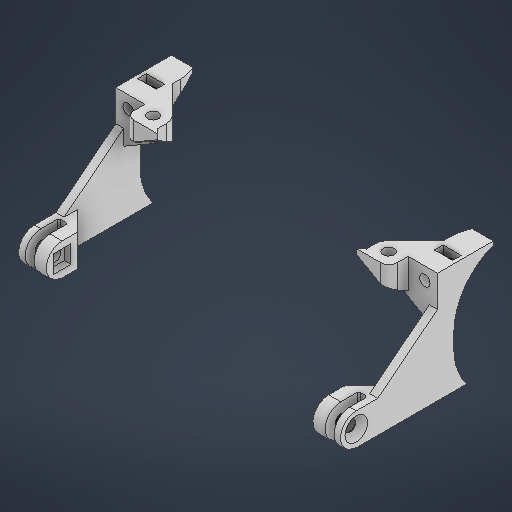
# Autodesk Inventor part: body-main
Saved by Autodesk Inventor 2025 (Build 290162000, 162)
## iProperties
Created: 2024-10-19
Part Number: body-main
Material: Všeobecné
Document SubType Name: Modeling
Designer: Simak
Density: 1 g/cm^3
Appearance: Výchozí
Author: Simak
Autodesk Inventor part; units mm, degrees
ref_plane "YZ Plane" through (0, 0, 0) normal (1, 0, 0) x (0, 1, 0)
ref_plane "XZ Plane" through (0, 0, 0) normal (0, 1, 0) x (-1, 0, 0)
ref_plane "XY Plane" through (0, 0, 0) normal (0, 0, 1) x (1, 0, 0)
sketch "Náčrt1" plane through (0, 0, 0) normal (1, 0, 0) x (0, 1, 0)
  circle A0 centre (5, 0) radius 5 construction
  line L0 (10, 0) -> (10, -6.8) construction
  line L1 (9.85, -6.6099) -> (24.35, -24.9833)
  line L2 (0, 0) -> (0, -39.0132)
  line L3 (24.35, -24.9833) -> (34, -24.9833)
  line L4 (34, -24.9833) -> (34, -42.1726)
  circle A1 centre (13.5, -48.5) radius 16.5 construction
  line L5 (10, -5) -> (0, -5) construction
  line L6 (15.5, -30) -> (11.5, -30)
  arc A2 (11.5, -30) -> (0, -34.0086) centre (11.5, -48.5) ccw
  arc A3 (32.8843, -42.1726) -> (15.5, -30) centre (15.5, -48.5) ccw
  line L7 (32.8843, -42.1726) -> (34, -45.238) construction
  line L8 (32.8843, -42.1726) -> (34, -42.1726)
  circle A4 centre (5, 0) radius 4.85
  line L9 (9.85, 0) -> (9.85, -6.6099)
  line L10 (0, 0) -> (0.2955, 1.1791)
  point P0 (13.5, -65)
  point P1 (13.5, -30)
  dimension "d0" = 10
  dimension "d1" = 33
  dimension "d3" = 3
  dimension "d4" = 65
  dimension "d5" = 128.28
  dimension "d6" = 34
  dimension "d7" = 9.65
  dimension "d8" = 6.8
  dimension "d9" = 4
  dimension "d10" = 2
  dimension "d11" = 18.5
  dimension "d13" = 70
  dimension "d14" = 9.7
  constraints: 23 end point, 10 point on circle, 8 tangent, 7 point on line, 5 centre point, 4 perpendicular, 2 horizontal, 2 vertical, 2 vertical alignment, 1 coincident, 1 equal radius, 1 midpoint
  measures "d0" diameter of A0
  measures "d1" diameter of A1
  measures "d3" distance edge to line of A1 L2
  measures "d4" vertical distance of A1.start A0.centre
  measures "d5" angle of L1 L5
  measures "d6" distance between parallel lines of L4 L2
  measures "d7" distance of L1.end L3.end
  measures "d8" vertical distance of A0.centre L0.end
  measures "d9" distance of L6.start L6.end
  measures "d10" distance edge to line of A1 L6
  measures "d11" radius of A2
  measures "d13" angle of L7 L3
  measures "d14" diameter of A4
extrude "Vysunutí1" add sketch "Náčrt1" along normal blind 49.5
sketch "Náčrt2" plane through (0, 0, -34.0086) normal (0, -1, 0) x (1, 0, 0)
  line L0 (0, 38.8586) -> (49.5, 38.8586) projected
  line L1 (49.5, 34.0086) -> (49.5, 38.8586) projected
  line L2 (49.5, 34.0086) -> (49.5, 35.1877) projected
  line L3 (49.5, 35.1877) -> (49.5, 34.0086) projected
  line L4 (49.5, 34.0086) -> (49.5, 0) projected
  line L5 (49.5, 0) -> (49.5, 4.0086) projected
  line L6 (49.5, 4.0086) -> (49.5, -8.164) projected
  line L7 (49.5, -8.164) -> (49.5, 9.0253) projected
  line L8 (49.5, 9.0253) -> (49.5, 27.3987) projected
  line L9 (49.5, 27.3987) -> (49.5, 34.0086) projected
  line L10 (0, 34.0086) -> (0, 35.1877) projected
  line L11 (0, 27.3987) -> (0, 34.0086) projected
  line L12 (0, 9.0253) -> (0, 27.3987) projected
  line L13 (0, -8.164) -> (0, 9.0253) projected
  line L14 (0, 4.0086) -> (0, -8.164) projected
  line L15 (0, 0) -> (0, 4.0086) projected
  line L16 (0, 34.0086) -> (0, 0) projected
  line L17 (0, 35.1877) -> (0, 34.0086) projected
  line L18 (0, 34.0086) -> (0, 38.8586) projected
  line L19 (0, -8.164) -> (49.5, -8.164) projected
  line L20 (47, 38.8586) -> (47, -8.164)
  dimension "d17" = 2.5
  constraints: 2 end point, 2 point on line, 1 perpendicular
  measures "d17" distance between parallel lines of L8 L20
extrude "Vysunutí2" cut sketch "Náčrt2" against normal through all contours L0 L20 L19 L13 L12 L11 L10 L18
sketch "Náčrt3" plane through (49.5, 0, -34.0086) normal (0, -1, 0) x (1, 0, 0)
  line L0 (-2.5, 38.8586) -> (0, 38.8586) projected
  line L1 (0, 34.0086) -> (0, 35.1877) projected
  line L2 (0, 35.1877) -> (0, 34.0086) projected
  line L3 (0, 34.0086) -> (0, 0) projected
  line L4 (0, 0) -> (0, 4.0086) projected
  line L5 (0, 4.0086) -> (0, -8.164) projected
  line L6 (0, -8.164) -> (0, 9.0253) projected
  line L7 (0, 9.0253) -> (0, 27.3987) projected
  line L8 (0, 27.3987) -> (0, 34.0086) projected
  line L9 (0, 34.0086) -> (0, 38.8586) projected
  line L10 (-2.5, 0) -> (-2.5, 4.0086) projected
  line L11 (-2.5, 34.0086) -> (-2.5, 0) projected
  line L12 (-2.5, 35.1877) -> (-2.5, 34.0086) projected
  line L13 (-2.5, 34.0086) -> (-2.5, 35.1877) projected
  line L14 (-2.5, 27.3987) -> (-2.5, 34.0086) projected
  line L15 (-2.5, 9.0253) -> (-2.5, 27.3987) projected
  line L16 (-2.5, -8.164) -> (-2.5, 9.0253) projected
  line L17 (-2.5, 4.0086) -> (-2.5, -8.164) projected
  line L18 (-2.5, 34.0086) -> (-2.5, 38.8586) projected
  line L19 (-2.5, -8.164) -> (0, -8.164) projected
  line L20 (-2, 38.8586) -> (-2, 29.0086)
  line L21 (-49.5, 29.1586) -> (-49.5, 38.8586) projected
  line L22 (-49.5, 29.0086) -> (-49.5, 39.0086) construction
  line L23 (-2, 29.0086) -> (-4.75, 29.0086)
  line L24 (-4.75, 29.0086) -> (-4.75, 38.8586)
  line L25 (-6.5, 38.8586) -> (-6.5, 27.2231)
  line L26 (-4.75, 38.8586) -> (-6.5, 38.8586)
  line L27 (-6.5, 27.2231) -> (-2.5, 23.2231)
  line L28 (-2, 29.0086) -> (-2.5, 28.5086)
  line L29 (-4.75, 29.0086) -> (-4.25, 28.5086)
  line L30 (-4.25, 28.5086) -> (-2.5, 28.5086)
  point P0 (-49.5, 34.0086)
  point P1 (-49.5, 34.0086)
  point P2 (-2.5, 29.0086)
  dimension "d20" = 2
  dimension "d21" = 2.75
  dimension "d22" = 6.5
  dimension "d23" = 45
  dimension "d24" = 2.5
  dimension "d25" = 45
  constraints: 18 end point, 3 horizontal, 3 perpendicular, 3 point on line, 2 horizontal alignment, 1 vertical
  measures "d20" distance between parallel lines of L9 L20
  measures "d21" distance of L20.end L23.end
  measures "d22" distance between parallel lines of L3 L25
  measures "d23" angle of L15 L27
  measures "d24" distance from line of L23.end L27
  measures "d25" angle of L14 L28
extrude "Vysunutí3" cut sketch "Náčrt3" against normal up to surface (9.85 mm away) contours L0 L20 L23 L11 L12 L18 | L28 L11 L23
extrude "Vysunutí4" add sketch "Náčrt3" against normal up to surface (9.85 mm away) contours L11 L27 L25 L26 L24 L29 L30
sketch "Náčrt4" plane through (49.5, 0, 0) normal (1, 0, 0) x (0, 0, -1)
  line L0 (5, 9.85) -> (-4.85, 9.85) projected
  line L1 (-4.85, 0) -> (-4.85, 9.85) projected
  line L2 (5, 0) -> (-4.85, 0) projected
  line L3 (5, 0) -> (5, 9.85) projected
  arc A0 (0, 9.85) -> (-1.1791, 0.2955) centre (0, 5) ccw projected
  line L4 (-1.1791, 0.2955) -> (0, 0) projected
  line L5 (0, 0) -> (34.0086, 0) projected
  arc A1 (30, 11.5) -> (34.0086, 0) centre (48.5, 11.5) ccw projected
  line L6 (30, 11.5) -> (30, 15.5) projected
  arc A2 (42.1726, 32.8843) -> (30, 15.5) centre (48.5, 15.5) ccw projected
  line L7 (42.1726, 32.8843) -> (42.1726, 34) projected
  line L8 (42.1726, 34) -> (24.9833, 34) projected
  line L9 (24.9833, 34) -> (24.9833, 24.35) projected
  line L10 (24.9833, 24.35) -> (6.6099, 9.85) projected
  line L11 (6.6099, 9.85) -> (0, 9.85) projected
  point P0 (-4.85, 5)
extrude "Vysunutí5" cut sketch "Náčrt4" against normal through all contours A0 L1 L0 | A0 L4 L2 L1
sketch "Náčrt5" plane through (49.5, 0, 0) normal (1, 0, 0) x (0, 0, -1)
  arc A0 (0, 9.85) -> (-1.1791, 0.2955) centre (0, 5) ccw projected
  point P0 (0, 0)
  constraints: 1 coincident
hole "Díra1" at (49.5, 5, 0) direction (-1, 0, 0) diameter 3.4 end through all countersink diameter 7 countersink angle 90
sketch "Náčrt6" plane through (43, 0, -6.7855) normal (-1, 0, 0) x (0, 0, 1)
  line L0 (4.0355, 7.75) -> (9.5355, 7.75)
  line L1 (9.5355, 7.75) -> (9.5355, 2.25)
  line L2 (9.5355, 2.25) -> (4.0355, 2.25)
  line L3 (4.0355, 2.25) -> (4.0355, 7.75)
  circle A0 centre (6.7855, 5) radius 3.5 projected
  line L4 (4.0355, 7.75) -> (6.7855, 5) construction
  line L5 (6.7855, 5) -> (9.5355, 7.75) construction
  line L6 (4.0355, 2.25) -> (6.7855, 5) construction
  circle A1 centre (6.7855, 5) radius 1.7 projected
  arc A2 (7.9646, 0.2955) -> (6.7855, 9.85) centre (6.7855, 5) ccw projected
  line L7 (6.7855, 9.85) -> (0, 9.85) projected
  line L8 (0, 0) -> (0, 9.85) projected
  line L9 (6.7855, 0) -> (0, 0) projected
  line L10 (6.7855, 0) -> (7.9646, 0.2955) projected
  dimension "d39" = 5.5
  constraints: 14 end point, 5 perpendicular, 2 parallel, 1 horizontal
  measures "d39" distance of L1.end L2.end
extrude "Vysunutí6" add sketch "Náčrt6" along normal blind 2 contours A0 L0 | L3 A0 | A0 L1 | L2 A0 | L10 L9 L8 L7 A2
sketch "Náčrt7" plane through (49.5, 9.85, 0) normal (0, 1, 0) x (1, 0, 0)
  line L0 (-8.5, 0) -> (-8.5, 6.7855) projected
  line L1 (-6.5, 6.7855) -> (-8.5, 6.7855) projected
  line L2 (-6.5, 6.7855) -> (-2.5, 10.7855) projected
  line L3 (-6.5, 6.7855) -> (-8.5, 4.7855)
  point P0 (-49.5, 0)
  constraints: 2 end point, 1 collinear, 1 point on line
extrude "Vysunutí7" cut sketch "Náčrt7" against normal through all
sketch "Náčrt8" plane through (49.5, 24.35, -24.9833) normal (0, 0, 1) x (1, 0, 0)
  circle A0 centre (-3.875, 5.775) radius 1.65
  line L0 (0, 9.65) -> (0, 0) projected
  line L1 (-2.5, 9.65) -> (0, 9.65) projected
  circle A1 centre (-3.875, 5.775) radius 3.875
  line L2 (-7.75, 3.85) -> (-2.5, -0.1301)
  line L3 (-2.5, 9.65) -> (-2.5, 0) projected
  line L4 (-2.5, 0) -> (-2.5, -14.5) projected
  line L5 (-3.875, 9.65) -> (-2.5, 9.65)
  line L6 (-7.75, 3.85) -> (-7.75, 5.775)
  point P0 (-49.5, -24.35)
  point P1 (-2.5, 9.3978)
  point P2 (0, 5.775)
  point P3 (-2.5, 2.1522)
  point P4 (-6.216, 2.6871)
  point P5 (-6.216, 2.6871)
  dimension "d44" = 3.875
  dimension "d45" = 3.875
  dimension "d46" = 3.3
  dimension "d77" = 5.8
  constraints: 6 end point, 4 tangent, 2 centre point, 2 point on circle, 1 coincident, 1 horizontal alignment, 1 point on line, 1 vertical, 1 vertical alignment
  measures "d44" distance from line of L0 A0.centre
  measures "d45" distance from line of L1 A0.centre
  measures "d46" diameter of A0
  measures "d77" distance from line of L2.start L1
extrude "Vysunutí8" add sketch "Náčrt8" against normal up to surface contours L3 A0 | A0 L3 A1 | A1 L5 L3 | L3 L4 L2 A1 | L2 L6 A1 round surface about axis through (0, 15.5, -48.5) along (1, 0, 0) radius 18.5 far side no picked at (-3.5043, 5.7082) picked at (-6.0124, 3.508)
extrude "Vysunutí9" cut sketch "Náčrt8" against normal through all contours A0 L3 | L3 A0
sketch "Náčrt9" plane through (49.5, 34, -24.9833) normal (0, 1, 0) x (1, 0, 0)
  line L0 (-5.525, 0) -> (-5.525, 12.1871) projected
  line L1 (-2.225, 0) -> (-2.225, 12.1871) projected
  line L2 (-7.75, 0) -> (-7.75, 12.1871) projected
  spline S0 degree 7 poles (-3.875, 23.5167) (-4.2595, 22.6766) (-4.6432, 21.8383) (-5.0232, 20.9998) (-5.3966, 20.1601) (-5.7592, 19.3189) (-6.1055, 18.4772) (-6.6646, 17.0171) (-6.8881, 16.3994) (-7.0958, 15.7818) (-7.284, 15.1633) (-7.4474, 14.545) (-7.5778, 13.9297) (-7.687, 13.1584) (-7.707, 12.9949) (-7.7236, 12.8319) (-7.7365, 12.6695) (-7.7454, 12.5078) (-7.75, 12.3469) (-7.75, 12.1871) knots 0 0 0 0 0 0 0 0 0.51596 0.51596 0.51596 0.51596 0.51596 0.51596 0.897167 0.897167 0.897167 0.897167 0.897167 0.897167 1 1 1 1 1 1 1 1 projected
  line L3 (-2.5, 23.5167) -> (-3.875, 23.5167) projected
  line L4 (-2.5, 17.1893) -> (-2.5, 23.5167) projected
  line L5 (-2.5, 17.1893) -> (-2.5, 12.1871)
  line L6 (-7.75, 12.1871) -> (-2.5, 12.1871)
  line L7 (-2.5, 17.1893) -> (-6.5956, 17.1893)
  point P0 (-49.5, -24.9833)
  point P1 (-5.8125, 8.8451)
  point P2 (-2.5, 8.6438)
  constraints: 6 end point, 2 horizontal, 1 vertical, 2 other
extrude "Vysunutí10" cut sketch "Náčrt9" against normal up to next contours L3 L4 L7 S0
ref_plane "Pracovní rovina1" through (49.5, 24.35, -30.7333) normal (0, 0, 1) x (1, 0, 0)
sketch "Náčrt10" plane through (49.5, 24.35, -30.7333) normal (0, 0, 1) x (1, 0, 0)
  arc A0 (-3.875, 9.65) -> (-7.75, 5.775) centre (-3.875, 5.775) ccw projected
  line L0 (-3.875, 9.65) -> (0, 9.65) projected
  circle A1 centre (-3.875, 5.775) radius 1.65 projected
  line L1 (-2.5, 0) -> (-2.5, -0.1301) projected
  line L2 (-2.5, 0) -> (0, 0) projected
  line L3 (0, 9.65) -> (0, 0) projected
  line L4 (-3.875, 9.65) -> (0, 9.65) projected
  arc A2 (-3.875, 9.65) -> (-7.75, 5.775) centre (-3.875, 5.775) ccw projected
  line L5 (-3.875, 2.5418) -> (-6.675, 4.1584)
  line L6 (-6.675, 4.1584) -> (-6.675, 7.3916)
  line L7 (-6.675, 7.3916) -> (-3.875, 9.0082)
  line L8 (-3.875, 9.0082) -> (-1.075, 7.3916)
  line L9 (-1.075, 7.3916) -> (-1.075, 4.1584)
  line L10 (-1.075, 4.1584) -> (-3.875, 2.5418)
  line L11 (-6.675, 7.3916) -> (-6.675, 8.4537)
  line L12 (-1.075, 7.3916) -> (-1.075, 9.65)
  line L13 (-7.75, 5.775) -> (-7.75, 3.85) projected
  line L14 (-7.75, 3.85) -> (-2.5, -0.1301) projected
  point P0 (-49.5, -24.35)
  point P1 (-1.075, 9.65)
  point P2 (-6.675, 8.4537)
  point P3 (-2.5, 2.1522)
  dimension "d61" = 5.6
  constraints: 16 end point, 1 coincident, 1 parallel, 1 point on circle, 1 point on line, 1 vertical, 1 vertical alignment, 13 other
  measures "d61" distance between parallel lines of L9 L6
extrude "Vysunutí11" cut sketch "Náčrt10" against normal blind 2.65 contours L0 L12 L8 L7 L11 A0 | L7 L8 L9 L10 L5 L6 | A1
sketch "Náčrt11" plane through (49.5, 34, -24.9833) normal (0, 1, 0) x (1, 0, 0)
  line L0 (-89.5, 39.5167) -> (-9.5, 39.5167) construction
  line L1 (-9.5, 39.5167) -> (-9.5, -5.4833) construction
  line L2 (-9.5, -5.4833) -> (-89.5, -5.4833) construction
  line L3 (-89.5, -5.4833) -> (-89.5, 39.5167) construction
  line L4 (-6.675, 8.4) -> (-3.875, 8.4) projected
  line L5 (-3.875, 8.4) -> (-3.875, 17.1893) projected
  spline S0 degree 7 poles (-6.5956, 17.1893) (-6.8005, 16.6342) (-6.9933, 16.0803) (-7.1719, 15.5262) (-7.3336, 14.9718) (-7.4738, 14.4179) (-7.5867, 13.8669) (-7.687, 13.1584) (-7.707, 12.9949) (-7.7236, 12.8319) (-7.7365, 12.6695) (-7.7454, 12.5078) (-7.75, 12.3469) (-7.75, 12.1871) knots 0 0 0 0 0 0 0 0 0.768736 0.768736 0.768736 0.768736 0.768736 0.768736 1 1 1 1 1 1 1 1 projected
  line L6 (-3.875, 0) -> (-7.75, 0) projected
  line L7 (-3.875, 0) -> (-3.875, 5.75) projected
  line L8 (-3.875, 5.75) -> (-6.675, 5.75) projected
  line L9 (-6.675, 5.75) -> (-6.675, 8.4) projected
  line L10 (-3.875, 17.1893) -> (-6.5956, 17.1893) projected
  line L11 (-6.675, 5.75) -> (-3.875, 5.75) projected
  line L12 (-3.875, 5.75) -> (-3.875, 8.4) projected
  line L13 (-3.875, 8.4) -> (-6.675, 8.4) projected
  line L14 (-6.675, 5.75) -> (-6.675, 8.4) projected
  line L15 (-7.75, 0) -> (-7.75, 12.1871) projected
  circle A0 centre (-13.25, -1.7333) radius 1.7
  line L16 (-9, 0) -> (-9, -3.4)
  line L17 (0, 17.1893) -> (0, 0) projected
  arc A1 (-11.5, -5.9) -> (-9, -3.4) centre (-11.5, -3.4) ccw
  line L18 (-11.5, -5.9) -> (-13.25, -5.9)
  line L19 (-7.75, 0) -> (-9, 0)
  line L20 (-7.75, 9.6593) -> (-16.1963, 1.213)
  arc A2 (-16.1963, 1.213) -> (-13.25, -5.9) centre (-13.25, -1.7333) ccw
  line L21 (-13.25, -5.9) -> (-17.4167, -5.9)
  line L22 (-17.4167, -5.9) -> (-17.4167, -1.7333)
  line L23 (-18.8667, -5.9) -> (-17.4167, -4.45)
  line L24 (-18.8667, -5.9) -> (-17.4167, -5.9)
  point P0 (-49.5, -24.9833)
  point P1 (-49.5, 40.0167)
  point P2 (-49.5, 39.5167)
  dimension "d64" = 80
  dimension "d65" = 45
  dimension "d66" = 0.5
  dimension "d81" = 3.4
  dimension "d82" = 3.75
  dimension "d83" = 3.75
  dimension "d84" = 9
  dimension "d85" = 2.5
  dimension "d87" = 5.9
  dimension "d88" = 45
  dimension "d90" = 135
  dimension "d91" = 1.45
  constraints: 25 end point, 6 tangent, 5 point on circle, 3 centre point, 3 horizontal, 3 perpendicular, 3 point on line, 2 parallel, 1 coincident, 1 horizontal alignment, 1 midpoint, 1 vertical, 1 vertical alignment, 1 other
  measures "d64" distance of L0.start L0.end
  measures "d65" distance of L0.end L1.end
  measures "d66" distance from line of L0 point (-49.5, 40.017)
  measures "d81" diameter of A0
  measures "d82" distance from line of L2 A0.centre
  measures "d83" distance from line of A0.centre L1
  measures "d84" distance between parallel lines of L17 L16
  measures "d85" radius of A1
  measures "d87" distance between parallel lines of L6 L18
  measures "d88" angle of L15 L20
  measures "d90" angle of L22 L23
  measures "d91" distance of L23.start L21.end
extrude "Vysunutí12" add sketch "Náčrt11" against normal blind 5.8 contours L19 L16 A1 L18 A2 L20 L15 | A2 L21 L22 | L22 L24 L23
extrude "Vysunutí13" add sketch "Náčrt11" against normal up to next contours L9 L8 L7 L6 L15 S0 L10 L5 L4
sketch "Náčrt12" plane through (49.5, 28.2, -24.9833) normal (0, -1, 0) x (1, 0, 0)
  circle A0 centre (-13.25, 1.7333) radius 1.7 projected
  line L0 (-13.25, 4.9087) -> (-10.5, 3.321)
  line L1 (-10.5, 3.321) -> (-10.5, 0.1456)
  line L2 (-10.5, 0.1456) -> (-13.25, -1.4421)
  line L3 (-13.25, -1.4421) -> (-16, 0.1456)
  line L4 (-16, 0.1456) -> (-16, 3.321)
  line L5 (-16, 3.321) -> (-13.25, 4.9087)
  point P0 (-49.5, 24.9833)
  dimension "d92" = 5.5
  constraints: 12 end point, 1 coincident, 1 vertical alignment, 13 other
  measures "d92" distance between parallel lines of L1 L4
extrude "Vysunutí14" cut sketch "Náčrt12" against normal blind 2.6
sketch "Náčrt14" plane through (32.0833, 34, -23.25) normal (-1, 0, 0) x (0, 0, 1)
  line L0 (-3.1754, -5.8) -> (-1.5877, -5.8) projected
  line L1 (-1.5877, -5.8) -> (1.5877, -5.8) projected
  line L2 (1.5877, -5.8) -> (3.1754, -5.8) projected
  line L3 (3.1754, -5.8) -> (1.5877, -5.8) projected
  line L4 (1.5877, -5.8) -> (-1.5877, -5.8) projected
  line L5 (-1.5877, -5.8) -> (-3.1754, -5.8) projected
  line L6 (-1.7333, -5.8) -> (-11.3926, -5.8) projected
  line L7 (-1.7333, -5.8) -> (1.6667, -5.8) projected
  line L8 (1.6667, -5.8) -> (4.1667, -5.8) projected
  line L9 (4.1667, -5.8) -> (2.7167, -5.8) projected
  line L10 (2.7167, -5.8) -> (0, -5.8) projected
  line L11 (0, -5.8) -> (-2.9463, -5.8) projected
  line L12 (-2.9463, -5.8) -> (-11.3926, -5.8) projected
  arc A0 (-8.934, -9.7801) -> (-11.7979, -5.8) centre (-25.25, -18.5) ccw projected
  line L13 (-11.3926, -5.8) -> (-11.7979, -5.8) projected
  line L14 (-1.7333, -5.8) -> (-1.7333, -9.7801) projected
  line L15 (-1.7333, -9.65) -> (16.6401, -24.15) projected
  line L16 (4.1667, -5.8) -> (2.7167, -5.8) projected
  line L17 (4.1667, -5.8) -> (-7.6991, -12.6507)
  arc A1 (-6.75, -18.5) -> (-8.934, -9.7801) centre (-25.25, -18.5) ccw projected
  line L18 (4.1667, 0) -> (4.1667, -5.8) projected
  point P0 (23.25, -34)
  point P1 (-1.7333, -9.2064)
  dimension "d100" = 60
  constraints: 2 end point, 1 point on circle
  measures "d100" angle of L18 L17
extrude "Vysunutí15" add sketch "Náčrt14" against normal up to surface (8.4167 mm away) contours L0 L1 L2 L8 L17 L14
sketch "Náčrt15" plane through (32.0833, 24.7936, -24.9833) normal (0, 0, -1) x (-1, 0, 0)
  line L0 (-8.4167, 3.4064) -> (-8.4167, 0) projected
  line L1 (0, 0) -> (-8.4167, 0) projected
  line L2 (0, 3.4064) -> (0, 0) projected
  line L3 (0, 3.4064) -> (-0.3776, 3.4064) projected
  line L4 (-1.6689, 3.4064) -> (-0.3776, 3.4064) projected
  line L5 (-1.6689, 3.4064) -> (-6.6645, 3.4064) projected
  line L6 (-8.4167, 3.4064) -> (-6.6645, 3.4064) projected
  line L7 (-1.2204, 3.4064) -> (-9.6667, 3.4064) projected
  line L8 (-9.6667, 3.4064) -> (-14.9167, -0.5737) projected
  line L9 (-14.9167, -9.2936) -> (-14.9167, -0.5737) projected
  line L10 (0, 3.4064) -> (-14.9167, -5.2058)
  point P0 (32.0833, -24.7936)
  point P1 (-5.9, 0)
  dimension "d103" = 60
  constraints: 2 end point, 1 point on line
  measures "d103" angle of L2 L10
extrude "Vysunutí16" add sketch "Náčrt15" along normal up to surface contours L6 L5 L4 L3 L10 L1 L0 | L0 L1 L10 L9 L8 L7 round surface about axis through (0, 15.5, -48.5) along (1, 0, 0) radius 18.5 far side no
extrude "Vysunutí17" cut sketch "Náčrt15" against normal through all contours L10 L2 L1
sketch "Náčrt16" plane through (49.5, 34, -24.9833) normal (0, 1, 0) x (1, 0, 0)
  line L0 (-6.675, 8.4) -> (-1.075, 8.4) projected
  line L1 (-1.075, 8.4) -> (-1.075, 5.75) projected
  line L2 (-1.075, 5.75) -> (-6.675, 5.75) projected
  line L3 (-6.675, 5.75) -> (-6.675, 8.4) projected
  circle A0 centre (-13.25, -1.7333) radius 1.7 projected
  line L4 (-6.5956, 17.1893) -> (0, 17.1893) projected
  line L5 (-7.75, 12.1871) -> (-7.75, 9.6593) projected
  line L6 (-7.75, 9.6593) -> (-16.1963, 1.213) projected
  arc A1 (-16.1963, 1.213) -> (-17.4167, -1.7333) centre (-13.25, -1.7333) ccw projected
  line L7 (-17.4167, -1.7333) -> (-17.4167, -4.45) projected
  line L8 (-17.4167, -4.45) -> (-18.8667, -5.9) projected
  line L9 (-18.8667, -5.9) -> (-11.5, -5.9) projected
  arc A2 (-11.5, -5.9) -> (-9, -3.4) centre (-11.5, -3.4) ccw projected
  line L10 (-9, -3.4) -> (-9, 0) projected
  line L11 (-9, 0) -> (0, 0) projected
  line L12 (0, 17.1893) -> (0, 0) projected
  arc A3 (-16.1963, 1.213) -> (-17.4167, -1.7333) centre (-13.25, -1.7333) ccw projected
  line L13 (-16.1963, 1.213) -> (-7.75, 9.6593) projected
  line L14 (-7.75, 9.6593) -> (-7.75, 10.0646) projected
  line L15 (-7.75, 10.0646) -> (-17.4167, 10.0646) projected
  line L16 (-17.4167, -1.7333) -> (-17.4167, 10.0646) projected
  arc A4 (-11.5, -5.9) -> (-9, -3.4) centre (-11.5, -3.4) ccw projected
  line L17 (-11.5, -5.9) -> (-9, -5.9) projected
  line L18 (-9, -5.9) -> (-9, -3.4) projected
  point P0 (-49.5, -24.9833)
  point P1 (-9, -3.4)
  point P2 (-11.5, -5.9)
  constraints: 1 other
extrude "Vysunutí18" cut sketch "Náčrt16" against normal through all contours L5 L6 A1 L16 L15 | A2 L18 L17
extrude "Vysunutí19" cut sketch "Náčrt12" along normal up to next contours A0 | L0 L1 L2 L3 L4 L5
sketch "Náčrt17" plane through (41.75, 27.7565, -34.6426) normal (-0.7071068, 0, -0.7071068) x (-0.7071068, 0, 0.7071068)
  line L0 (3.1179, -8.1687) -> (8.953, -3.4043) projected
  line L1 (8.953, -3.4043) -> (20.7989, 6.2678)
  line L2 (12.7667, 3.0435) -> (15.0121, 3.0435) projected
  line L3 (9.6995, 3.0435) -> (12.7667, 3.0435) projected
  line L4 (8.8777, 3.0435) -> (9.6995, 3.0435) projected
  line L5 (11.123, 3.0435) -> (8.8777, 3.0435) projected
  line L6 (14.1902, 3.0435) -> (11.123, 3.0435) projected
  line L7 (15.0121, 3.0435) -> (14.1902, 3.0435) projected
  line L8 (10.2449, 3.0435) -> (13.6449, 3.0435) projected
  line L9 (14.1902, -0.1288) -> (11.123, -1.0455) projected
  line L10 (12.7667, -0.3745) -> (15.0121, -0.3745) projected
  line L11 (14.7919, -0.7999) -> (14.1902, -0.1288) projected
  line L12 (17.8375, 0.4435) -> (14.7919, -0.7999) projected
  line L13 (18.8628, 0.4435) -> (16.8122, 0.4435) projected
  line L14 (18.8628, 6.2435) -> (18.8628, 0.4435) projected
  point P0 (54.0177, -27.7565)
  point P1 (18.8628, 4.687)
  point P2 (12.257, -0.7066)
  point P3 (13.3684, -0.3745)
  point P4 (14.4105, -0.3745)
  constraints: 2 end point, 1 collinear
extrude "Vysunutí20" cut sketch "Náčrt17" against normal through all
mirror "Zrcadlit1" about plane through (0, 5, 0) normal (-1, 0, 0)
equation "\"d45\" = d44"
equation "\"d83\" = d82"
